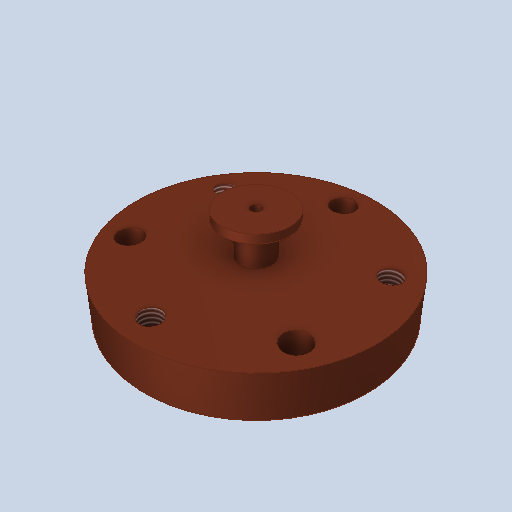
# Autodesk Inventor part: RodHolder-2023-1
Saved by Autodesk Inventor 2026 (Build 300175050, 175E)
## iProperties
Created: 2018-11-21
Part Number: RodHolder-2023-1
Material: Copper
Document SubType Name: Modeling
Designer: schanen
Density: 8.94 g/cm^3
Appearance: Copper - Satin
Mass: 30.6882 g
Surface Area: 22.6953 cm^2
Volume: 3.43268 cm^3
Author: schanen
Autodesk Inventor part; units mm, degrees
ref_plane "YZ Plane" through (0, 0, 0) normal (1, 0, 0) x (0, 1, 0)
ref_plane "XZ Plane" through (0, 0, 0) normal (0, 1, 0) x (-1, 0, 0)
ref_plane "XY Plane" through (0, 0, 0) normal (0, 0, 1) x (1, 0, 0)
sketch "Sketch1" plane through (0, 0, 0) normal (1, 0, 0) x (0, 1, 0)
  line L0 (0, 7.5) -> (0, 15)
  line L1 (0, 15) -> (5, 15)
  line L2 (5, 15) -> (5, 2)
  line L3 (5, 2) -> (9, 2)
  line L4 (9, 2) -> (9, 4)
  line L5 (9, 4) -> (10, 4)
  line L6 (10, 4) -> (10, 0.65)
  line L7 (10, 0.65) -> (3, 0.65)
  line L8 (3, 0.65) -> (3, 7.5)
  line L9 (3, 7.5) -> (0, 7.5)
  line L10 (-2, 0) -> (12, 0) projected
  point P0 (0, 0)
  dimension "d0" = 7.5
  dimension "d1" = 0.65
  dimension "d2" = 4
  dimension "d3" = 2
  dimension "d4" = 15
  dimension "d5" = 5
  dimension "d6" = 4
  dimension "d7" = 1
  dimension "d34" = 3
  constraints: 20 end point, 9 perpendicular, 1 vertical, 1 vertical alignment
  measures "d0" distance between parallel lines of L10 L9
  measures "d1" distance between parallel lines of L10 L7
  measures "d2" distance between parallel lines of L10 L5
  measures "d3" distance between parallel lines of L10 L3
  measures "d4" distance between parallel lines of L10 L1
  measures "d5" distance of L0.end L1.end
  measures "d6" distance of L2.end L3.end
  measures "d7" distance of L4.end L5.end
  measures "d34" distance of L8.end L0.start
revolve "Revolution1" add sketch "Sketch1" angle 360 about axis through (0, -10, 0) along (0, 1, 0)
sketch "Sketch2" plane through (0, 0, 0) normal (0, -1, 0) x (1, 0, 0)
  point P0 (0, 0)
  point P1 (0, -12)
  dimension "d10" = 12
  measures "d10" distance of point (0, 0) point (0, -12)
hole "Hole1" at (0, 0, -12) direction (0, 1, 0) diameter 3 end through all
pattern_circular "Circular Pattern1" count 3 over 360 about axis through (0, 2.5, 0) along (0, 1, 0) of "Hole1"
sketch "Sketch3" plane through (0, 0, 0) normal (0, -1, 0) x (1, 0, 0)
  circle A0 centre (0, 0) radius 12 construction
  circle A1 centre (0, -12) radius 1.5 projected
  point P0 (-10.3923, -6)
  dimension "d21" = 24
  dimension "d22" = 60
  constraints: 1 coincident, 3 other
hole "Hole2" at (-10.3923, 0, -6) direction (0, 1, 0) diameter 2.459 end through all thread size "M3x0.5" class "6H" standard "ANSI Metric M Profile"
pattern_circular "Circular Pattern2" count 3 over 360 about axis through (0, 2.5, 0) along (0, 1, 0) of "Hole2"
sketch "Sketch4" plane through (0, 3, 0) normal (0, -1, 0) x (1, 0, 0)
  point P0 (0, 0)
  point P1 (0, 0)
  constraints: 1 coincident
hole "Hole3" at (0, 3, 0) direction (0, 1, 0) diameter 3.2 depth 5 tip angle 118
body "Solid1"
